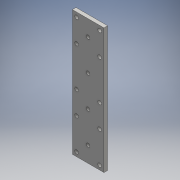
# Autodesk Inventor part: CouplingHeadSilicone_Base
Saved by Autodesk Inventor 2016 (Build 200138000, 138)
## iProperties
Created: 2015-12-21
Part Number: CouplingHeadSilicone_Base
Material: Generic
Document SubType Name: Modeling
Designer: m2memari
Density: 1 g/cm^3
Appearance: Default
Author: m2memari
Autodesk Inventor part; units mm, degrees
ref_plane "YZ Plane" through (0, 0, 0) normal (1, 0, 0) x (0, 1, 0)
ref_plane "XZ Plane" through (0, 0, 0) normal (0, 1, 0) x (-1, 0, 0)
ref_plane "XY Plane" through (0, 0, 0) normal (0, 0, 1) x (1, 0, 0)
sketch "Sketch1" plane through (0, 0, 0) normal (0, 1, 0) x (-1, 0, 0)
  circle A0 centre (0, 0) radius 21.4121 construction
  circle A1 centre (0, 0) radius 16.9043 construction
  circle A2 centre (0, 0) radius 3.175
  circle A3 centre (0, 0) radius 22.4121 construction
  circle A4 centre (0, -54.0936) radius 3.175
  circle A5 centre (0, -108.1872) radius 3.175
  circle A6 centre (0, -162.2808) radius 3.175
  circle A7 centre (0, -54.0936) radius 20.2851 construction
  circle A8 centre (0, -54.0936) radius 21.2851 construction
  circle A9 centre (0, -108.1872) radius 19.6089 construction
  circle A10 centre (0, -108.1872) radius 20.6089 construction
  circle A11 centre (0, -162.2808) radius 19.1582 construction
  circle A12 centre (0, -162.2808) radius 20.1582 construction
  line L0 (27.4121, 27.4121) -> (-27.4121, 27.4121)
  line L1 (-27.4121, 27.4121) -> (-27.4121, -189.6929)
  line L2 (-27.4121, -189.6929) -> (27.4121, -189.6929)
  line L3 (27.4121, -189.6929) -> (27.4121, 27.4121)
  circle A13 centre (-19.9121, 19.9121) radius 3.175
  circle A14 centre (19.9121, 19.9121) radius 3.175
  line L4 (0, 0) -> (-27.4121, 0) construction
  circle A15 centre (-19.9121, -19.9121) radius 3.175
  circle A16 centre (19.9121, -19.9121) radius 3.175
  line L5 (0, -54.0936) -> (-27.4121, -54.0936) construction
  circle A17 centre (19.9121, -88.2752) radius 3.175
  circle A18 centre (-19.9121, -88.2752) radius 3.175
  line L6 (0, -108.1872) -> (-27.4121, -108.1872) construction
  circle A19 centre (19.9121, -128.0993) radius 3.175
  circle A20 centre (-19.9121, -128.0993) radius 3.175
  line L7 (0, -162.2808) -> (-27.4121, -162.2808) construction
  circle A21 centre (19.9121, -182.1929) radius 3.175
  line L8 (0, -162.2808) -> (0, -189.6929) construction
  circle A22 centre (-19.9121, -182.1929) radius 3.175
  dimension "d1" = 42.8241
  dimension "d2" = 33.8085
  dimension "d4" = 6.35
  dimension "d11" = 44.8241
  dimension "d12" = 6.35
  dimension "d13" = 6.35
  dimension "d14" = 6.35
  dimension "d15" = 54.0936
  dimension "d16" = 54.0936
  dimension "d17" = 54.0936
  dimension "d18" = 40.5702
  dimension "d19" = 42.5702
  dimension "d20" = 39.2179
  dimension "d21" = 41.2179
  dimension "d22" = 38.3163
  dimension "d23" = 40.3163
  dimension "d31" = 27.4121
  dimension "d32" = 27.4121
  dimension "d33" = 27.4121
  dimension "d34" = 27.4121
  dimension "d37" = 6.35
  dimension "d38" = 7.5
  dimension "d39" = 7.5
  dimension "d40" = 6.35
  dimension "d41" = 7.5
  dimension "d50" = 6.35
  dimension "d51" = 7.5
  constraints: 23 centre point, 18 end point, 10 coincident, 7 symmetric about line, 5 perpendicular, 4 point on line, 4 vertical alignment, 2 parallel, 1 horizontal, 1 horizontal alignment, 1 midpoint, 7 other
  measures "d1" diameter of A0
  measures "d2" diameter of A1
  measures "d4" diameter of A2
  measures "d11" diameter of A3
  measures "d12" diameter of A4
  measures "d13" diameter of A5
  measures "d14" diameter of A6
  measures "d15" distance of A4.centre point (0, 0)
  measures "d16" distance of A4.centre A5.centre
  measures "d17" distance of A6.centre A5.centre
  measures "d18" diameter of A7
  measures "d19" diameter of A8
  measures "d20" diameter of A9
  measures "d21" diameter of A10
  measures "d22" diameter of A11
  measures "d23" diameter of A12
  measures "d31" distance from line of L3 L4.start
  measures "d32" distance from line of L1 L4.start
  measures "d33" distance from line of L0 L4.start
  measures "d34" distance from line of L2 L7.start
  measures "d37" diameter of A13
  measures "d38" distance from line of L0 A13.centre
  measures "d39" distance from line of L1 A13.centre
  measures "d40" diameter of A14
  measures "d41" distance from line of L3 A14.centre
  measures "d50" diameter of A21
  measures "d51" distance from line of L2 A21.centre
extrude "Extrusion4" add sketch "Sketch1" along normal blind 6.39
equation "\"d1\" = 0.95 * d0"
equation "\"d2\" = 0.75 * d0"
equation "\"d12\" = d4"
equation "\"d13\" = d4"
equation "\"d14\" = d4"
equation "\"d15\" = 1.2 * d0"
equation "\"d16\" = d15"
equation "\"d17\" = d15"
equation "\"d18\" = 0.9 * d0"
equation "\"d20\" = 0.87 * d0"
equation "\"d22\" = 0.85 * d0"
equation "\"d32\" = d31"
equation "\"d33\" = d31"
equation "\"d34\" = d31"
equation "\"d54\" = WoodThickness"
equation "\"d0\" = 45.078"
equation "\"WoodThickness\" = 6.39"
body "Solid4"
